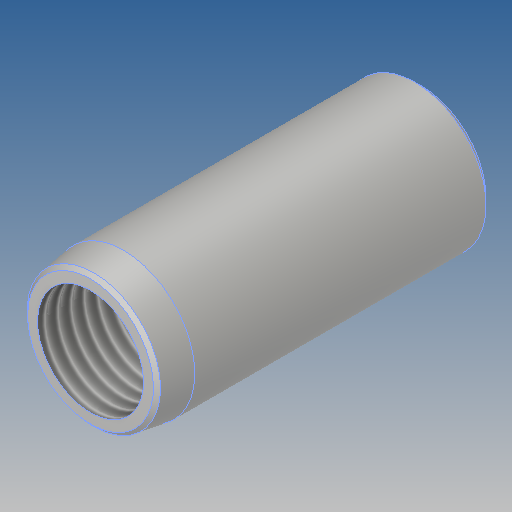
# Autodesk Inventor part: support_douille
Saved by Autodesk Inventor 2019 (Build 230136000, 136)
## iProperties
Created: 2019-03-25
Part Number: support_douille
Material: Aluminium 6061
Document SubType Name: Modeling
Designer: theor
Density: 2.7 g/cm^3
Appearance: Aluminium - Plat
Mass: 22.6287 g
Surface Area: 60.9293 cm^2
Volume: 8.381 cm^3
Author: theor
Autodesk Inventor part; units mm, degrees
ref_plane "XZ Plane" through (0, 0, 0) normal (0, 1, 0) x (-1, 0, 0)
ref_plane "XY Plane" through (0, 0, 0) normal (0, 0, 1) x (1, 0, 0)
sketch "Esquisse1" plane through (0, 0, 0) normal (1, 0, 0) x (0, 1, 0)
  line L0 (0, 0) -> (0, 17.1522)
  line L1 (8, 50) -> (8, 36)
  line L2 (8, 36) -> (6, 36)
  line L3 (6, 36) -> (6, 30)
  line L4 (6, 30) -> (8.25, 23.8182)
  line L5 (8.25, 23.8182) -> (8.25, 1)
  line L6 (8.25, 1) -> (9.25, 0)
  line L7 (9.25, 0) -> (9.75, 0)
  line L8 (8, 50) -> (10, 50)
  line L9 (10, 50) -> (10.75, 45)
  line L10 (10.75, 45) -> (10.75, 1)
  line L11 (10.75, 1) -> (9.75, 0)
  dimension "d0" = 160
  dimension "d1" = 6
  dimension "d2" = 14
  dimension "d4" = 16
  dimension "d6" = 16.5
  dimension "d8" = 1
  dimension "d9" = 1
  dimension "d10" = 30
  dimension "d11" = 2
  dimension "d12" = 2
  dimension "d13" = 21.5
  dimension "d14" = 2.5
  dimension "d15" = 5
  dimension "d19" = 1
  dimension "d20" = 1
  dimension "d48" = 2.75
  dimension "d49" = 4.75
  constraints: 25 end point, 5 vertical, 3 horizontal, 1 horizontal alignment
  measures "d0" angle of L3 L4
  measures "d1" distance of L2.end L3.end
  measures "d2" distance of L1.start L1.end
  measures "d4" diameter of L1 L0
  measures "d6" diameter of L5 L0
  measures "d8" horizontal distance of L5.end L6.end
  measures "d9" horizontal distance of L5.end L6.end
  measures "d10" vertical distance of L3.end L6.end
  measures "d11" distance of L1.start L8.end
  measures "d12" distance between parallel lines of L3 L1
  measures "d13" diameter of L10 L0
  measures "d14" distance between parallel lines of L10 L5
  measures "d15" vertical distance of L8.end L9.end
  measures "d19" horizontal distance of L10.end L7.end
  measures "d20" horizontal distance of L10.end L7.end
  measures "d48" distance between parallel lines of L10 L1
  measures "d49" distance between parallel lines of L10 L3
revolve "Révolution1" add sketch "Esquisse1" angle 360 about axis through (0, 0, 0) along (0, 0, 1)
thread "Filetage1" size "M16x2" class "6H" standard "ISO Metric profile" full length
ref_plane "Plan de construction2" through (14, 0, 0) normal (1, 0, 0) x (0, 1, 0)
chamfer "Chanfrein4" distance 0.5 angle 45 1 edges at (0, -10, 50)
